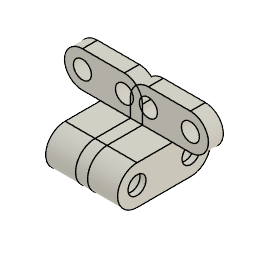
ServoSupport_v8 (Autodesk Fusion 360 design; units mm, degrees)
Autodesk Fusion 360 part; units mm, degrees
sketch "Sketch1" plane through (0, 0, 0) normal (1, 0, 0) x (0, 1, 0)
  circle A0 centre (-4.5, 0) radius 1.5
  circle A1 centre (4.5, 0) radius 3.24
  circle A2 centre (-4.5, 0) radius 2.1
  line L0 (4.5, 0) -> (-4.5, 0) construction
  circle A3 centre (-4.5, 0) radius 3.24
  circle A4 centre (4.5, 0) radius 2.1
  circle A5 centre (4.5, 0) radius 1.5
  line L1 (-4.5, 3.24) -> (4.5, 3.24)
  line L2 (4.5, -3.24) -> (-4.5, -3.24)
  line L3 (2.6474, 3.24) -> (2.6474, 9.24) construction
  line L4 (1.3974, 9.24) -> (3.8974, 9.24)
  line L5 (3.8974, 9.24) -> (3.8974, 3.24)
  line L6 (1.3974, 9.24) -> (1.3974, 3.24)
  dimension "d2" = 4.2
  dimension "d3" = 9
  dimension "d4" = 4.2
  dimension "d6" = 3
  dimension "d7" = 3
  dimension "d8" = 6
  dimension "d9" = 2.5
  constraint coincident A1.centre L0.start
  constraint coincident A0.centre A2.centre
  constraint concentric A2 A3
  constraint concentric A1 A4
  constraint concentric A4 A5
  constraint concentric A0 A2
  constraint horizontal L0
  constraint midpoint origin L0
  constraint coincident A3 L1.start
  constraint coincident A1 L1.end
  constraint tangent A1 L1
  constraint coincident A1 L2.start
  constraint coincident A3 L2.end
  constraint tangent A3 L2
  constraint horizontal L2
  constraint tangent A3 L1
  constraint tangent A1 L2
  constraint perpendicular L1 L3
  constraint midpoint L3.end L4
  constraint perpendicular L3 L4
  constraint coincident L1 L5.end
  constraint perpendicular L1 L5
  constraint coincident L1 L6.end
  constraint perpendicular L1 L6
  measures "d2" diameter of A4
  measures "d3" distance of A0.centre A1.centre
  measures "d4" diameter of A2
  measures "d6" diameter of A5
  measures "d7" diameter of A0
  measures "d8" distance of L3.start L3.end
  measures "d9" distance of L4.start L4.end
extrude "Extrude1" add sketch "Sketch1" against normal blind 1 contours A1 | A1 A3 L1 L2 | L1 L4 L5 L6 | A3 makes body 1
extrude "Extrude2" add sketch "Sketch1" along normal blind 6 contours A1 | A1 A3 L1 L2 | L1 L4 L5 L6 | A3 bodies 1
extrude "Extrude3" add sketch "Sketch1" along normal blind 12 contours L1 L4 L5 L6 bodies 1
sketch "Sketch2" plane through (0, 1.3974, 0) normal (0, -1, 0) x (1, 0, 0)
  line L0 (-1, 3.24) -> (6, 3.24)
  line L1 (12, 9.24) -> (-1, 9.24)
  line L2 (12, 3.24) -> (12, 9.24)
  line L3 (-1, 9.24) -> (-1, 3.24)
  circle A0 centre (9, 6.24) radius 1.5
  circle A1 centre (2, 6.24) radius 1.5
  line L4 (-1, 6.24) -> (12, 6.24) construction
  line L5 (6, 3.24) -> (12, 3.24)
  dimension "d17" = 3
  dimension "d18" = 3
  dimension "d31" = 3
  dimension "d32" = 3
  constraint midpoint L2 L4.end
  constraint coincident A0.centre L4
  constraint coincident A1.centre L4
  constraint coincident L3 L4.start
  constraint midpoint L3 L4.start
  measures "d17" diameter of A0
  measures "d18" diameter of A1
  measures "d31" distance of L2 A0.centre
  measures "d32" distance of L3 A1.centre
extrude "Extrude4" cut sketch "Sketch2" against normal blind 4 contours A0 | A1 bodies 1
sketch "Sketch3" plane through (6, 0, 0) normal (1, 0, 0) x (0, 1, 0)
  line L0 (1.3974, 3.24) -> (-4.5, 3.24)
  arc A0 (-4.5, 3.24) -> (-4.5, -3.24) centre (-4.5, 0) ccw
  line L1 (-4.5, -3.24) -> (4.5, -3.24)
  arc A1 (4.5, -3.24) -> (4.5, 3.24) centre (4.5, 0) ccw
  line L2 (4.5, 3.24) -> (3.8974, 3.24)
  circle A2 centre (-4.5, 0) radius 2.1
  circle A3 centre (4.5, 0) radius 2.1
  circle A4 centre (4.5, 0) radius 1.5
  circle A5 centre (-4.5, 0) radius 1.5
  line L3 (3.8974, 3.24) -> (1.3974, 3.24)
  dimension "d27" = 3
  dimension "d28" = 3
  constraint concentric A1 A4
  constraint concentric A0 A5
  measures "d27" diameter of A4
  measures "d28" diameter of A5
extrude "Extrude5" add sketch "Sketch3" against normal blind 1 contours A2 | A3 bodies 1
fillet "Fillet3" radius 3 3 edges at (12, 2.6474, 3.24) (12, 2.6474, 9.24) (-1, 2.6474, 9.24) on bodies 1
mirror "Mirror1" about plane through (0, 0, 0) normal (1, 0, 0) of bodies 1 makes body 2
